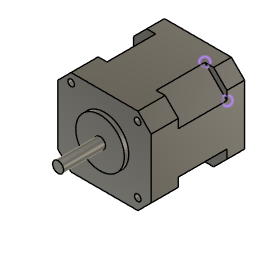
stepper v1 (Autodesk Fusion 360 design; units mm, degrees)
Autodesk Fusion 360 part; units mm, degrees
sketch "Sketch1" plane through (0, 0, 0) normal (0, 0, 1) x (1, 0, 0)
  line L0 (21.15, -21.15) -> (-21.15, -21.15)
  line L1 (-21.15, -21.15) -> (-21.15, 21.15)
  line L2 (-21.15, 21.15) -> (21.15, 21.15)
  line L3 (21.15, 21.15) -> (21.15, -21.15)
  line L4 (21.15, -21.15) -> (-21.15, 21.15) construction
  line L5 (-21.15, -21.15) -> (21.15, 21.15) construction
  dimension "d3" = 42.3
  dimension "d4" = 42.3
  constraint horizontal L0
  constraint perpendicular L0 L1
  constraint parallel L0 L2
  constraint parallel L1 L3
  constraint coincident L4 origin
  constraint coincident L5 origin
  measures "d3" distance of L1.end L2.end
  measures "d4" distance of L0.end L1.end
extrude "Extrude1" add sketch "Sketch1" along normal blind 39
chamfer "Chamfer1" distance 6 angle 45 4 edges at (-21.15, 0, 39) (21.15, 0, 39) (21.15, 0, 0) (-21.15, 0, 0)
sketch "Sketch2" plane through (0, -21.15, 0) normal (0, -1, 0) x (1, 0, 0)
  line L0 (-21.15, 6) -> (-15.15, 0)
  line L1 (-15.15, 0) -> (15.15, 0)
  line L2 (15.15, 0) -> (21.15, 6)
  line L3 (21.15, 6) -> (21.15, 33)
  line L4 (21.15, 33) -> (15.15, 39)
  line L5 (15.15, 39) -> (-15.15, 39)
  line L6 (-15.15, 39) -> (-21.15, 33)
  line L7 (-21.15, 33) -> (-21.15, 6)
  circle A0 centre (0, 20) radius 2.5
  dimension "d8" = 5
  measures "d8" diameter of A0
extrude "Extrude2" add sketch "Sketch2" along normal blind 21 contours A0
sketch "Sketch3" plane through (0, -21.15, 0) normal (0, -1, 0) x (1, 0, 0)
  circle A0 centre (0, 20) radius 2.5
  line L0 (-21.15, 6) -> (-15.15, 0)
  line L1 (-15.15, 0) -> (15.15, 0)
  line L2 (15.15, 0) -> (21.15, 6)
  line L3 (21.15, 6) -> (21.15, 33)
  line L4 (21.15, 33) -> (15.15, 39)
  line L5 (15.15, 39) -> (-15.15, 39)
  line L6 (-15.15, 39) -> (-21.15, 33)
  line L7 (-21.15, 33) -> (-21.15, 6)
  circle A1 centre (0, 20) radius 11
  dimension "d11" = 22
  constraint concentric A0 A1
  measures "d11" diameter of A1
extrude "Extrude3" add sketch "Sketch3" along normal blind 2 contours A1
sketch "Sketch4" plane through (0, -21.15, 0) normal (0, -1, 0) x (1, 0, 0)
  circle A0 centre (0, 20) radius 11
  line L0 (-21.15, 6) -> (-15.15, 0)
  line L1 (-15.15, 0) -> (15.15, 0)
  line L2 (15.15, 0) -> (21.15, 6)
  line L3 (21.15, 6) -> (21.15, 33)
  line L4 (21.15, 33) -> (15.15, 39)
  line L5 (15.15, 39) -> (-15.15, 39)
  line L6 (-15.15, 39) -> (-21.15, 33)
  line L7 (-21.15, 33) -> (-21.15, 6)
  circle A1 centre (-15.0778, 34.9879) radius 1.5
  circle A2 centre (15.0778, 5.0121) radius 1.5
  circle A3 centre (14.9957, 34.9599) radius 1.5
  circle A4 centre (-15.1592, 5.2464) radius 1.5
  dimension "d14" = 3
  dimension "d16" = 360
  dimension "d17" = 3
  dimension "d18" = 3
  measures "d14" diameter of A1
  measures "d17" diameter of A3
  measures "d18" diameter of A4
extrude "Extrude4" cut sketch "Sketch4" against normal blind 4.5 contours A1 | A2 | A3 | A4
sketch "Sketch5" plane through (0, 21.15, 0) normal (0, 1, 0) x (-1, 0, 0)
  line L0 (15.15, 0) -> (21.15, 6)
  line L1 (21.15, 6) -> (21.15, 33)
  line L2 (21.15, 33) -> (15.15, 39)
  line L3 (15.15, 39) -> (-15.15, 39)
  line L4 (-15.15, 39) -> (-21.15, 33)
  line L5 (-21.15, 33) -> (-21.15, 6)
  line L6 (-21.15, 6) -> (-15.15, 0)
  line L7 (-15.15, 0) -> (15.15, 0)
  line L8 (-11.15, 39) -> (-21.15, 29)
  line L9 (-21.15, 29) -> (-21.15, 39)
  line L10 (-11.15, 39) -> (-21.15, 39)
  dimension "d21" = 10
  dimension "d22" = 10
  constraint coincident L3 L8.start
  constraint coincident L5 L8.end
  constraint parallel L4 L8
  constraint parallel L5 L9
  constraint perpendicular L9 L10
  measures "d21" distance of L5 L8.start
  measures "d22" distance of L3 L8.end
extrude "Extrude5" cut sketch "Sketch5" against normal blind 22 from surface at -8 contours L3 L4 L5 L8 L9 L10 | L4 L9 L10
sketch "Sketch6" plane through (0, 21.15, 0) normal (0, 1, 0) x (-1, 0, 0)
  line L0 (15.15, 0) -> (21.15, 6)
  line L1 (21.15, 6) -> (21.15, 33)
  line L2 (21.15, 33) -> (15.15, 39)
  line L3 (15.15, 39) -> (-15.15, 39)
  line L4 (-15.15, 39) -> (-21.15, 33)
  line L5 (-21.15, 33) -> (-21.15, 6)
  line L6 (-21.15, 6) -> (-15.15, 0)
  line L7 (-15.15, 0) -> (15.15, 0)
  line L8 (11.15, 39) -> (21.15, 29)
  line L9 (11.15, 39) -> (21.15, 39)
  line L10 (21.15, 29) -> (21.15, 39)
  dimension "d26" = 10
  dimension "d27" = 10
  constraint coincident L3 L8.start
  constraint coincident L1 L8.end
  constraint parallel L3 L9
  constraint perpendicular L9 L10
  measures "d26" distance of L1 L8.start
  measures "d27" distance of L3 L8.end
extrude "Extrude6" cut sketch "Sketch6" against normal blind 22 from surface at -8 contours L1 L2 L3 L8 L9 L10 | L2 L9 L10
sketch "Sketch7" plane through (0, 21.15, 0) normal (0, 1, 0) x (-1, 0, 0)
  line L0 (15.15, 0) -> (21.15, 6)
  line L1 (21.15, 6) -> (21.15, 33)
  line L2 (21.15, 33) -> (15.15, 39)
  line L3 (15.15, 39) -> (-15.15, 39)
  line L4 (-15.15, 39) -> (-21.15, 33)
  line L5 (-21.15, 33) -> (-21.15, 6)
  line L6 (-21.15, 6) -> (-15.15, 0)
  line L7 (-15.15, 0) -> (15.15, 0)
  line L8 (21.15, 10) -> (11.15, 0)
  line L9 (11.15, 0) -> (21.15, 0)
  line L10 (21.15, 10) -> (21.15, 0)
  dimension "d31" = 10
  dimension "d32" = 10
  constraint coincident L1 L8.start
  constraint coincident L7 L8.end
  constraint parallel L7 L9
  constraint perpendicular L9 L10
  measures "d31" distance of L7 L8.start
  measures "d32" distance of L1 L8.end
extrude "Extrude7" cut sketch "Sketch7" against normal blind 22 from surface at -8 contours L0 L1 L7 L8 L9 L10 | L0 L9 L10
sketch "Sketch8" plane through (0, 21.15, 0) normal (0, 1, 0) x (-1, 0, 0)
  line L0 (15.15, 0) -> (21.15, 6)
  line L1 (21.15, 6) -> (21.15, 33)
  line L2 (21.15, 33) -> (15.15, 39)
  line L3 (15.15, 39) -> (-15.15, 39)
  line L4 (-15.15, 39) -> (-21.15, 33)
  line L5 (-21.15, 33) -> (-21.15, 6)
  line L6 (-21.15, 6) -> (-15.15, 0)
  line L7 (-15.15, 0) -> (15.15, 0)
  line L8 (-11.15, 0) -> (-21.15, 10)
  line L9 (-11.15, 0) -> (-21.15, 0)
  line L10 (-21.15, 10) -> (-21.15, 0)
  dimension "d36" = 10
  dimension "d37" = 10
  constraint coincident L7 L8.start
  constraint coincident L5 L8.end
  constraint parallel L7 L9
  constraint perpendicular L9 L10
  measures "d36" distance of L5 L8.start
  measures "d37" distance of L7 L8.end
extrude "Extrude8" cut sketch "Sketch8" against normal blind 22 from surface at -8 contours L5 L6 L7 L8 L9 L10 | L6 L9 L10
sketch "Sketch9" plane through (0, 13.15, 0) normal (0, -1, 0) x (1, 0, 0)
  line L0 (21.15, 33) -> (15.15, 39)
  line L1 (15.15, 39) -> (11.15, 39)
  line L2 (21.15, 29) -> (21.15, 33)
sketch "Sketch10" plane through (0, 13.15, 0) normal (0, -1, 0) x (1, 0, 0)
sketch "Sketch11" plane through (0, 13.15, 0) normal (0, -1, 0) x (1, 0, 0)
sketch "Sketch12" plane through (0, 13.15, 0) normal (0, -1, 0) x (1, 0, 0)
